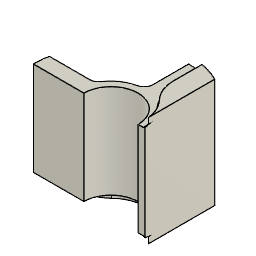
Pacifier Fixture (Autodesk Fusion 360 design; units mm, degrees)
part number: 2026-07-01-20-42-26-965
Autodesk Fusion 360 part; units mm, degrees
note: some values were not read from the file. Chosen so that the rebuilt part matches the saved one: which face or edge a step refers to.
sketch "Skizze1" plane through (0, 0, 0) normal (0, 0, 1) x (1, 0, 0)
  circle A0 centre (0, 0) radius 15.7
  circle A1 centre (0, 0) radius 19.7
  circle A2 centre (0, 0) radius 8.5
  circle A3 centre (0, 0) radius 45
  line L0 (0, -8.5) -> (-44.1899, -8.5)
  line L1 (0, 8.5) -> (-44.1899, 8.5)
  line L2 (0, 0) -> (0, 45)
  line L3 (8.5, 0) -> (8.5, 44.1899)
  line L4 (19.7, 0) -> (19.7, 40.4587)
  line L5 (-45, 0) -> (45, 0)
  dimension "d1" = 31.4
  dimension "d2" = 39.4
  dimension "d3" = 17
  dimension "d4" = 90
  constraint coincident A0.centre A1.centre
  constraint concentric A0 A2
  constraint concentric A0 A3
  constraint coincident A2 L0.start
  constraint coincident A3 L0.end
  constraint tangent A2 L0
  constraint horizontal L0
  constraint coincident A2 L1.start
  constraint coincident A3 L1.end
  constraint tangent A2 L1
  constraint parallel L0 L1
  constraint coincident A3 L2.end
  constraint vertical L2
  constraint coincident A2 L3.start
  constraint coincident A3 L3.end
  constraint tangent A2 L3
  constraint parallel L2 L3
  constraint coincident A1 L4.start
  constraint coincident A3 L4.end
  constraint tangent A1 L4
  constraint vertical L4
  constraint coincident A3 L5.start
  constraint coincident A3 L5.end
  constraint horizontal L5
  measures "d1" diameter of A0
  measures "d2" diameter of A1
  measures "d3" diameter of A2
  measures "d4" diameter of A3
extrude "Extrusion1" add sketch "Skizze1" along normal blind 9 contours A1 A3 L3 L4 | A1 A3 L2 L3 | A1 A3 L1 L2
extrude "Extrusion2" add sketch "Skizze1" along normal blind 54.4158 from surface at 4.5 contours A0 A1 L3 L5 | A0 A1 L2 L3 | A1 A3 L3 L4 | A0 A1 L1 L2 | A1 A3 L2 L3 | A0 A1 L1 L5 | A1 A3 L1 L5
extrude "Extrusion3" add sketch "Skizze1" along normal blind 4.5 from surface at 58.9158 contours A1 A3 L3 L4
move_face "Flächen versetzen1" offset -0.1 4 faces at (19.6784, 0.9228, 60.4158) (8.5, 26.5779, 60.4158) (-16.8362, 10.2289, 3) (-26.5779, 8.5, 1.5)
fillet "Abrundung1" radius 20 2 edges at (-17.8348, 8.6, 2.25) (8.6, 17.8348, 61.1658)
fillet "Abrundung2" radius 5 5 edges at (0, 32.35, 9) (-10.5033, 16.6664, 9) (-30.9809, 8.5, 9) (-17.7719, 8.5, 33.9579) (0, 19.7, 33.9579)
fillet "Abrundung3" radius 1 6 edges at (6.8008, 18.5954, 4.5) (-20.1761, 10.0604, 4.5) (-35.9244, 8.6, 4.5) (17.9578, 8.34, 58.9158) (10.0604, 20.1761, 58.9158) (8.6, 35.9244, 58.9158)
equation "d8 = ( 36.2376 * 1.75 ) * 1 mm - 9 mm"
named bodies: "Fixture"
